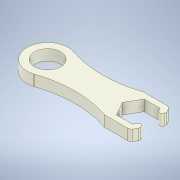
# Autodesk Inventor part: ShortLink
Saved by Autodesk Inventor 2022 (Build 260153000, 153)
## iProperties
Created: 2021-12-08
Part Number: ShortLink
Material: Genérico
Document SubType Name: Modeling
Designer: JK
Density: 1 g/cm^3
Appearance: Suave - Marfil
Author: JK
Autodesk Inventor part; units mm, degrees
ref_plane "YZ Plane" through (0, 0, 0) normal (1, 0, 0) x (0, 1, 0)
ref_plane "XZ Plane" through (0, 0, 0) normal (0, 1, 0) x (-1, 0, 0)
ref_plane "XY Plane" through (0, 0, 0) normal (0, 0, 1) x (1, 0, 0)
sketch "Boceto1" plane through (0, 0, 0) normal (0, 1, 0) x (-1, 0, 0)
  line L0 (6.2354, 0) -> (3.1177, -5.4)
  line L1 (3.1177, -5.4) -> (-3.1177, -5.4)
  line L2 (-3.1177, -5.4) -> (-6.2354, 0)
  line L3 (-6.2354, 0) -> (-3.1177, 5.4)
  line L4 (-3.1177, 5.4) -> (3.1177, 5.4)
  line L5 (3.1177, 5.4) -> (6.2354, 0)
  circle A0 centre (0, 0) radius 5.4
  line L6 (4.3879, 0) -> (2.1939, -3.8)
  line L7 (2.1939, -3.8) -> (-2.1939, -3.8)
  line L8 (-2.1939, -3.8) -> (-4.3879, 0)
  line L9 (-4.3879, 0) -> (-2.1939, 3.8)
  line L10 (-2.1939, 3.8) -> (2.1939, 3.8)
  line L11 (2.1939, 3.8) -> (4.3879, 0)
  dimension "d0" = 10.8
  dimension "d4" = 1.6
  constraints: 24 end point, 2 coincident, 1 centre point, 1 tangent, 18 other
  measures "d0" diameter of A0
  measures "d4" distance between parallel lines of L2 L8
extrude "Extrusión1" add sketch "Boceto1" along normal blind 3
sketch "Boceto2" plane through (0, 3, 0) normal (0, 1, 0) x (1, 0, 0)
  line L0 (8.9124, 8.7156) -> (4, 8.7156)
  line L1 (4, 8.7156) -> (4, -10.3861)
  line L2 (4, -10.3861) -> (8.9124, -10.3861)
  line L3 (8.9124, -10.3861) -> (8.9124, 8.7156)
  point P0 (0, 0)
  dimension "d22" = 4
  constraints: 8 end point, 2 parallel, 1 horizontal, 1 perpendicular
  measures "d22" distance from line of L1 point (0, 0)
extrude "Extrusión2" cut sketch "Boceto2" against normal through all
fillet "Empalme1" radius 1 4 edges at (3.1177, 1.5, -5.4) (3.1177, 1.5, 5.4) (-3.1177, 1.5, 5.4) (-3.1177, 1.5, -5.4)
fillet "Empalme2" radius 0.7 2 edges at (4, 1.5, -0.6718) (4, 1.5, 0.6718)
sketch "Boceto3" plane through (0, 3, 0) normal (0, 1, 0) x (1, 0, 0)
  line L0 (-23.3379, 5.4) -> (-4.3879, 5.4)
  line L1 (-4.3879, 5.4) -> (-4.3879, -5.4)
  line L2 (-4.3879, -5.4) -> (-23.3379, -5.4)
  line L3 (-23.3379, -5.4) -> (-23.3379, 5.4)
  line L4 (-23.3379, 5.4) -> (-4.3879, -5.4) construction
  line L5 (-4.3879, 5.4) -> (-23.3379, -5.4) construction
  line L6 (2.6938, -2.9342) -> (2.1939, -3.8) projected
  line L7 (2.1939, -3.8) -> (-2.1939, -3.8) projected
  line L8 (-2.1939, -3.8) -> (-4.3879, 0) projected
  line L9 (-4.3879, 0) -> (-2.1939, 3.8) projected
  line L10 (-2.1939, 3.8) -> (2.1939, 3.8) projected
  line L11 (2.1939, 3.8) -> (2.6938, 2.9342) projected
  arc A0 (3.4064, 4.9) -> (2.5403, 5.4) centre (2.5403, 4.4) ccw projected
  line L12 (2.5403, 5.4) -> (-2.5403, 5.4) projected
  arc A1 (-2.5403, 5.4) -> (-3.4064, 4.9) centre (-2.5403, 4.4) ccw projected
  line L13 (-3.4064, 4.9) -> (-6.2354, 0) projected
  line L14 (-6.2354, 0) -> (-3.4064, -4.9) projected
  arc A2 (-3.4064, -4.9) -> (-2.5403, -5.4) centre (-2.5403, -4.4) ccw projected
  line L15 (-2.5403, -5.4) -> (2.5403, -5.4) projected
  arc A3 (2.5403, -5.4) -> (3.4064, -4.9) centre (2.5403, -4.4) ccw projected
  line L16 (-4.3879, 5.4) -> (-0.8083, 5.4)
  line L17 (-0.8083, 5.4) -> (-0.8083, -5.4)
  line L18 (-0.8083, -5.4) -> (-4.3879, -5.4)
  line L19 (-4.3879, -5.4) -> (-4.3879, 5.4)
  circle A4 centre (-25, 0) radius 3.6
  circle A5 centre (-25, 0) radius 5.65
  line L20 (3.4064, -4.9) -> (4, -3.8718) projected
  line L21 (4, 3.8718) -> (3.4064, 4.9) projected
  line L22 (4, -3.8718) -> (4, -3.2842) projected
  line L23 (4, 3.2842) -> (4, 3.8718) projected
  arc A6 (4, -3.2842) -> (2.6938, -2.9342) centre (3.3, -3.2842) ccw projected
  arc A7 (2.6938, 2.9342) -> (4, 3.2842) centre (3.3, 3.2842) ccw projected
  point P0 (0, 0)
  point P1 (-13.8629, 0)
  point P2 (-13.8629, 0)
  point P3 (-13.8629, 0)
  point P4 (-2.5403, -5.4)
  point P5 (-2.5403, 5.4)
  point P6 (-23.3379, 5.4)
  point P7 (-2.8868, 4)
  point P8 (-4.3879, 3.2)
  point P9 (-4.3879, -3.2)
  point P10 (-23.3379, 5.4)
  point P11 (-0.8083, -3.8)
  point P12 (-0.8083, 3.8)
  point P13 (-0.8083, 5.4)
  dimension "d12" = 11.3
  dimension "d10" = 25
  dimension "d11" = 7.2
  constraints: 20 end point, 5 midpoint, 4 parallel, 2 horizontal, 2 horizontal alignment, 2 perpendicular, 1 centre point, 1 coincident, 1 collinear, 1 point on line, 3 other
  measures "d10" distance of point (0, 0) A4.centre
  measures "d11" diameter of A4
extrude "Extrusión3" add sketch "Boceto3" against normal up to surface (3 mm away) contours A5 L3 A4 | L0 L1 L13 L14 L2 A5 | L3 A4 A5 | L16 A1 L13 L1 | L1 L14 A2 L18
sketch "Boceto4" plane through (0, 3, 0) normal (0, 1, 0) x (1, 0, 0)
  arc A0 (-23.3379, 5.4) -> (-4, 5.4) centre (-13.669, 33.7991) ccw
  line L0 (-23.3379, -5.4) -> (2.5403, -5.4) projected
  arc A1 (-4, -5.4) -> (-23.3379, -5.4) centre (-13.669, -33.7991) ccw
  circle A2 centre (-25, 0) radius 3.6 projected
  line L1 (2.6938, -2.9342) -> (2.1939, -3.8) projected
  line L2 (2.1939, -3.8) -> (-2.1939, -3.8) projected
  line L3 (-2.1939, -3.8) -> (-4.3879, 0) projected
  line L4 (-4.3879, 0) -> (-2.1939, 3.8) projected
  line L5 (-2.1939, 3.8) -> (2.1939, 3.8) projected
  line L6 (2.1939, 3.8) -> (2.6938, 2.9342) projected
  arc A3 (3.4064, 4.9) -> (2.5403, 5.4) centre (2.5403, 4.4) ccw projected
  line L7 (2.5403, 5.4) -> (-23.3379, 5.4) projected
  arc A4 (-23.3379, 5.4) -> (-23.3379, -5.4) centre (-25, 0) ccw projected
  line L8 (-23.3379, -5.4) -> (2.5403, -5.4) projected
  arc A5 (2.5403, -5.4) -> (3.4064, -4.9) centre (2.5403, -4.4) ccw projected
  line L9 (3.4064, -4.9) -> (4, -3.8718) projected
  line L10 (4, 3.8718) -> (3.4064, 4.9) projected
  line L11 (4, 3.2842) -> (4, 3.8718) projected
  line L12 (4, -3.8718) -> (4, -3.2842) projected
  arc A6 (4, -3.2842) -> (2.6938, -2.9342) centre (3.3, -3.2842) ccw projected
  arc A7 (2.6938, 2.9342) -> (4, 3.2842) centre (3.3, 3.2842) ccw projected
  line L13 (2.5403, 5.4) -> (-23.3379, 5.4) projected
  point P0 (0, 0)
  point P1 (-4, 5.4)
  dimension "d16" = 4
  dimension "d18" = 30
  constraints: 4 point on circle, 2 centre point, 1 equal radius, 1 point on line, 1 vertical alignment
  measures "d16" horizontal distance of point (0, 0) A0.end
  measures "d18" radius of A0
extrude "Extrusión4" cut sketch "Boceto4" against normal through all contours L7 A0 | A1 L0
fillet "Empalme4" radius 3 2 edges at (-23.3379, 1.5, -5.4) (-23.3379, 1.5, 5.4)
